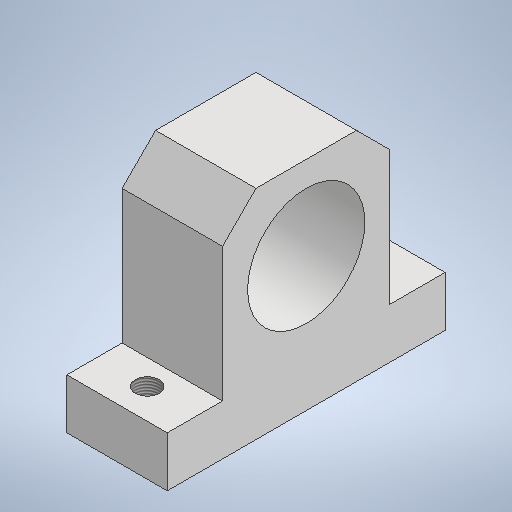
# Autodesk Inventor part: Pillow_block
Saved by Autodesk Inventor 2025.2 (Build 292293000, 293)
## iProperties
Created: 2025-02-20
Part Number: Pillow_block
Material: Generic
Document SubType Name: Modeling
Designer: Sergio Quintero
Density: 1 g/cm^3
Appearance: Default
Author: Sergio Quintero
Autodesk Inventor part; units mm, degrees
ref_plane "YZ Plane" through (0, 0, 0) normal (1, 0, 0) x (0, 1, 0)
ref_plane "XZ Plane" through (0, 0, 0) normal (0, 1, 0) x (-1, 0, 0)
ref_plane "XY Plane" through (0, 0, 0) normal (0, 0, 1) x (1, 0, 0)
sketch "Sketch1" plane through (0, 0, 0) normal (0, 1, 0) x (-1, 0, 0)
  line L0 (-15, -41.5) -> (15, -41.5)
  line L1 (15, -41.5) -> (15, 41.5)
  line L2 (15, 41.5) -> (-15, 41.5)
  line L3 (-15, 41.5) -> (-15, -41.5)
  line L4 (-15, -41.5) -> (15, 41.5) construction
  line L5 (15, -41.5) -> (-15, 41.5) construction
  point P0 (0, 0)
  dimension "d0" = 30
  dimension "d1" = 83
  constraints: 12 end point, 2 midpoint, 2 parallel, 1 horizontal, 1 perpendicular
  measures "d0" distance of L2.end L1.end
  measures "d1" distance of L1.end L0.end
extrude "Extrusion1" add sketch "Sketch1" along normal blind 15
sketch "Sketch2" plane through (0, 15, 0) normal (0, 1, 0) x (1, 0, 0)
  line L0 (-15, 41.5) -> (-15, -41.5) projected
  line L1 (15, 25) -> (-15, 25)
  line L2 (-15, 25) -> (-15, -25)
  line L3 (-15, -25) -> (15, -25)
  line L4 (15, -25) -> (15, 25)
  line L5 (15, 25) -> (-15, -25) construction
  line L6 (-15, 25) -> (15, -25) construction
  point P0 (0, 0)
  point P1 (-15, 25)
  dimension "d4" = 50
  constraints: 12 end point, 2 midpoint, 2 parallel, 1 horizontal, 1 perpendicular, 1 point on line
  measures "d4" distance of L2.end L1.end
extrude "Extrusion2" add sketch "Sketch2" along normal blind 50
chamfer "Chamfer1" distance 10 angle 45 2 edges at (0, 65, 25) (0, 65, -25)
sketch "Sketch3" plane through (0, 15, 0) normal (0, 1, 0) x (1, 0, 0)
  line L0 (-15, 41.5) -> (-15, 25) projected
  line L1 (15, 41.5) -> (-15, 41.5) projected
  point P0 (0, 0)
  point P1 (0, 32.5)
  point P2 (-15, 33.25)
  dimension "d10" = 15
  dimension "d11" = 9
  constraints: 1 midpoint
  measures "d10" horizontal distance of point (0, 32.5) point (-15, 33.25)
  measures "d11" distance from line of L1 point (0, 32.5)
hole "Hole1" at (0, 15, -32.5) direction (0, -1, 0) diameter 7.134 end through all thread size "M8x0.8" class "6H" standard "ISO Metric profile"
mirror "Mirror1" about plane through (0, 0, 0) normal (0, 0, 1) of "Hole1"
sketch "Sketch4" plane through (-15, 0, -41.5) normal (-1, 0, 0) x (0, 0, 1)
  circle A0 centre (41.5, 40) radius 17.5
  line L0 (26.5, 65) -> (56.5, 65) projected
  line L1 (66.5, 15) -> (66.5, 55) projected
  point P0 (41.5, 0)
  dimension "d19" = 35
  dimension "d20" = 25
  dimension "d21" = 25
  constraints: 1 centre point
  measures "d19" diameter of A0
  measures "d20" distance from line of A0.centre L0
  measures "d21" distance from line of A0.centre L1
extrude "Extrusion3" cut sketch "Sketch4" against normal blind 50
body "Solid1"
